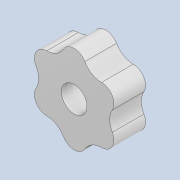
# Autodesk Inventor part: 1ギア接続部
Saved by Autodesk Inventor 2020.4 (Build 244396000, 396)
## iProperties
Created: 2021-04-23
Part Number: 1ギア接続部
Material: アルミニウム 2014-T4
Document SubType Name: Modeling
Designer: happy
Density: 2.8 g/cm^3
Appearance: サテン
Author: happy
Autodesk Inventor part; units mm, degrees
ref_plane "YZ Plane" through (0, 0, 0) normal (1, 0, 0) x (0, 1, 0)
ref_plane "XZ Plane" through (0, 0, 0) normal (0, 1, 0) x (-1, 0, 0)
ref_plane "XY Plane" through (0, 0, 0) normal (0, 0, 1) x (1, 0, 0)
sketch "スケッチ1" plane through (0, 0, 0) normal (0, 0, 1) x (1, 0, 0)
  circle A0 centre (45.6488, -28.0072) radius 8
  circle A1 centre (45.6488, -28.0072) radius 7 construction
  line L0 (45.6488, -21.0072) -> (51.7109, -24.5072) construction
  line L1 (51.7109, -24.5072) -> (51.7109, -31.5072) construction
  line L2 (51.7109, -31.5072) -> (45.6488, -35.0072) construction
  line L3 (45.6488, -35.0072) -> (39.5866, -31.5072) construction
  line L4 (39.5866, -31.5072) -> (39.5866, -24.5072) construction
  line L5 (39.5866, -24.5072) -> (45.6488, -21.0072) construction
  arc A2 (47.3808, -22.0072) -> (43.9167, -22.0072) centre (45.6488, -23.0072) ccw
  arc A3 (41.3186, -23.5072) -> (39.5866, -26.5072) centre (41.3186, -25.5072) ccw
  arc A4 (39.5866, -29.5072) -> (41.3186, -32.5072) centre (41.3186, -30.5072) ccw
  arc A5 (43.9167, -34.0072) -> (47.3808, -34.0072) centre (45.6488, -33.0072) ccw
  arc A6 (49.9789, -32.5072) -> (51.7109, -29.5072) centre (49.9789, -30.5072) ccw
  arc A7 (51.7109, -26.5072) -> (49.9789, -23.5072) centre (49.9789, -25.5072) ccw
  arc A8 (47.3808, -22.0072) -> (49.9789, -23.5072) centre (49.9789, -20.5072) ccw
  arc A9 (41.3186, -23.5072) -> (43.9167, -22.0072) centre (41.3186, -20.5072) ccw
  arc A10 (39.5866, -29.5072) -> (39.5866, -26.5072) centre (36.9885, -28.0072) ccw
  arc A11 (43.9167, -34.0072) -> (41.3186, -32.5072) centre (41.3186, -35.5072) ccw
  arc A12 (49.9789, -32.5072) -> (47.3808, -34.0072) centre (49.9789, -35.5072) ccw
  arc A13 (51.7109, -26.5072) -> (51.7109, -29.5072) centre (54.309, -28.0072) ccw
  circle A14 centre (45.6488, -28.0072) radius 5.6603 construction
  circle A15 centre (45.6488, -28.0072) radius 2.025
  point P0 (0, 0)
  point P1 (51.7109, -31.5072)
  point P2 (51.7109, -24.5072)
  point P3 (51.7109, -26.5072)
  point P4 (43.9167, -22.0072)
  point P5 (41.3186, -23.5072)
  point P6 (39.5866, -26.5072)
  dimension "d5" = 14
  dimension "d4" = 16
  dimension "d6" = 360
  dimension "d7" = 360
  dimension "d8" = 11.3205
  dimension "d9" = 3
  dimension "d10" = 2
  dimension "d13" = 4.05
  constraints: 30 point on circle, 15 centre point, 12 end point, 4 coincident, 2 point on line, 2 tangent, 1 vertical, 1 vertical alignment, 73 other
  measures "d4" diameter of A0
  measures "d8" diameter of A14
  measures "d9" radius of A8
  measures "d10" radius of A2
  measures "d13" diameter of A15
extrude "押し出し1" add sketch "スケッチ1" along normal blind 5 contours A8 A7 A13 A6 A12 A5 A11 A4 A10 A3 A9 A2
sketch "スケッチ2" plane through (0, 0, 5) normal (0, 0, 1) x (1, 0, 0)
  arc A0 (49.9789, -32.5072) -> (47.3808, -34.0072) centre (49.9789, -35.5072) ccw projected
  arc A1 (49.9789, -32.5072) -> (51.7109, -29.5072) centre (49.9789, -30.5072) ccw projected
  arc A2 (51.7109, -26.5072) -> (51.7109, -29.5072) centre (54.309, -28.0072) ccw projected
  arc A3 (51.7109, -26.5072) -> (49.9789, -23.5072) centre (49.9789, -25.5072) ccw projected
  arc A4 (47.3808, -22.0072) -> (49.9789, -23.5072) centre (49.9789, -20.5072) ccw projected
  arc A5 (47.3808, -22.0072) -> (43.9167, -22.0072) centre (45.6488, -23.0072) ccw projected
  arc A6 (41.3186, -23.5072) -> (43.9167, -22.0072) centre (41.3186, -20.5072) ccw projected
  arc A7 (41.3186, -23.5072) -> (39.5866, -26.5072) centre (41.3186, -25.5072) ccw projected
  arc A8 (39.5866, -29.5072) -> (39.5866, -26.5072) centre (36.9885, -28.0072) ccw projected
  arc A9 (39.5866, -29.5072) -> (41.3186, -32.5072) centre (41.3186, -30.5072) ccw projected
  arc A10 (43.9167, -34.0072) -> (41.3186, -32.5072) centre (41.3186, -35.5072) ccw projected
  arc A11 (43.9167, -34.0072) -> (47.3808, -34.0072) centre (45.6488, -33.0072) ccw projected
  circle A12 centre (45.6488, -28.0072) radius 2.025 projected
  arc A13 (41.3186, -23.5572) -> (39.6299, -26.4822) centre (41.3186, -25.5072) ccw
  arc A14 (41.3186, -23.5572) -> (43.96, -22.0322) centre (41.3186, -20.5072) ccw
  arc A15 (47.3375, -22.0322) -> (43.96, -22.0322) centre (45.6488, -23.0072) ccw
  arc A16 (47.3375, -22.0322) -> (49.9789, -23.5572) centre (49.9789, -20.5072) ccw
  arc A17 (51.6676, -26.4822) -> (49.9789, -23.5572) centre (49.9789, -25.5072) ccw
  arc A18 (51.6676, -26.4822) -> (51.6676, -29.5322) centre (54.309, -28.0072) ccw
  arc A19 (49.9789, -32.4572) -> (51.6676, -29.5322) centre (49.9789, -30.5072) ccw
  arc A20 (49.9789, -32.4572) -> (47.3375, -33.9822) centre (49.9789, -35.5072) ccw
  arc A21 (43.96, -33.9822) -> (47.3375, -33.9822) centre (45.6488, -33.0072) ccw
  arc A22 (43.96, -33.9822) -> (41.3186, -32.4572) centre (41.3186, -35.5072) ccw
  arc A23 (39.6299, -29.5322) -> (41.3186, -32.4572) centre (41.3186, -30.5072) ccw
  arc A24 (39.6299, -29.5322) -> (39.6299, -26.4822) centre (36.9885, -28.0072) ccw
  point P0 (0, 0)
  dimension "d14" = 0.05
  constraints: 24 point on circle, 12 centre point, 11 other
  measures "d14" radial gap between concentric circles of A8 A24
extrude "押し出し2" cut sketch "スケッチ2" against normal blind 10 contours A0 A11 A10 A9 A8 A7 A6 A5 A4 A3 A2 A1
